rpi_2_model_b (Autodesk Fusion 360 design; units mm, degrees)
Autodesk Fusion 360 part; units mm, degrees
sketch "Sketch1" plane through (0, 0, 0) normal (0, 0, 1) x (1, 0, 0)
  line L0 (0, -3) -> (-79, -3)
  line L1 (-82, 0) -> (-82, 50)
  line L2 (-79, 53) -> (0, 53)
  line L3 (3, 50) -> (3, 0)
  arc A0 (-79, 53) -> (-82, 50) centre (-79, 50) ccw
  arc A1 (-82, 0) -> (-79, -3) centre (-79, 0) ccw
  arc A2 (3, 50) -> (0, 53) centre (0, 50) ccw
  arc A3 (0, -3) -> (3, 0) centre (0, 0) ccw
  circle A4 centre (-78.5, 49.5) radius 1.375
  circle A5 centre (-78.5, 0.5) radius 1.375
  circle A6 centre (-20.5, 49.5) radius 1.375
  circle A7 centre (-20.5, 0.5) radius 1.375
  dimension "d1" = 3
  dimension "d2" = 85
  dimension "d3" = 56
  dimension "d4" = 49
  dimension "d5" = 0.5
  dimension "d6" = 0.5
  dimension "d7" = 2.75
  dimension "d8" = 2.75
  dimension "d9" = 3.5
  dimension "d10" = 2.75
  dimension "d11" = 2.75
  dimension "d12" = 58
  dimension "d13" = 58
  dimension "d14" = 49
  dimension "d15" = 49
  constraint horizontal L0
  constraint vertical L1
  constraint horizontal L2
  constraint vertical L3
  constraint tangent L1 A0
  constraint tangent L2 A0
  constraint tangent L0 A1
  constraint tangent L1 A1
  constraint equal A0 A1
  constraint tangent L2 A2
  constraint tangent L3 A2
  constraint equal A0 A2
  constraint tangent L0 A3
  constraint tangent L3 A3
  constraint equal A0 A3
  constraint coincident A3.centre origin
  measures "d1" radius of A0
  measures "d2" distance of L1 L3
  measures "d3" distance of L0 L2
  measures "d4" distance of A4.centre A5.centre
  measures "d5" vertical distance of A0.centre A4.centre
  measures "d6" vertical distance of A1.centre A5.centre
  measures "d7" diameter of A4
  measures "d8" diameter of A5
  measures "d9" distance of L1 A5.centre
  measures "d10" diameter of A7
  measures "d11" diameter of A6
  measures "d12" horizontal distance of A4.centre A6.centre
  measures "d13" horizontal distance of A4.centre A7.centre
  measures "d14" vertical distance of A4.centre A7.centre
  measures "d15" vertical distance of A5.centre A6.centre
extrude "Extrude1" add sketch "Sketch1" along normal blind 1.6
sketch "Sketch2" plane through (0, 0, 0) normal (0, 0, -1) x (1, 0, 0)
  circle A0 centre (-20.5, -49.5) radius 1.375
  circle A1 centre (-78.5, -0.5) radius 1.375
  circle A2 centre (-20.5, -0.5) radius 1.375
  circle A3 centre (-78.5, -49.5) radius 1.375
  arc A4 (-79, 3) -> (-82, 0) centre (-79, 0) ccw
  line L0 (-82, 0) -> (-82, -50)
  arc A5 (-82, -50) -> (-79, -53) centre (-79, -50) ccw
  line L1 (-79, -53) -> (0, -53)
  arc A6 (0, -53) -> (3, -50) centre (0, -50) ccw
  line L2 (3, -50) -> (3, 0)
  arc A7 (3, 0) -> (0, 3) centre (0, 0) ccw
  line L3 (0, 3) -> (-79, 3)
  line L4 (-67.4, -18.5) -> (-85.4, -18.5)
  line L5 (-85.4, -18.5) -> (-85.4, -33.1)
  line L6 (-85.4, -33.1) -> (-67.4, -33.1)
  line L7 (-67.4, -33.1) -> (-67.4, -18.5)
  dimension "d18" = 14.6
  dimension "d19" = 19.9
  dimension "d20" = 18
  dimension "d21" = 3.4
  constraint horizontal L4
  constraint vertical L5
  constraint horizontal L6
  constraint vertical L7
  measures "d18" distance of L4.end L5.end
  measures "d19" distance of L1 L6
  measures "d20" distance of L4.start L4.end
  measures "d21" distance of L0 L5
extrude "Extrude2" add sketch "Sketch2" along normal blind 1.4 contours L0 L4 L6 L7 | L0 L4 L5 L6
extrude "Extrude3" add 1 faces at (-36.7049, 22.8333, 0) along direction (0, 0, -1) blind 2.45
sketch "Sketch3" plane through (0, 0, 1.6) normal (0, 0, 1) x (-1, 0, 0)
  circle A0 centre (20.5, -49.5) radius 1.375
  circle A1 centre (78.5, -0.5) radius 1.375
  circle A2 centre (20.5, -0.5) radius 1.375
  circle A3 centre (78.5, -49.5) radius 1.375
  arc A4 (82, 0) -> (79, 3) centre (79, 0) ccw
  line L0 (79, 3) -> (0, 3)
  arc A5 (0, 3) -> (-3, 0) centre (0, 0) ccw
  line L1 (-3, 0) -> (-3, -50)
  arc A6 (-3, -50) -> (0, -53) centre (0, -50) ccw
  line L2 (0, -53) -> (79, -53)
  arc A7 (79, -53) -> (82, -50) centre (79, -50) ccw
  line L3 (82, -50) -> (82, 0)
  line L4 (31.5, -9.5) -> (25.5, -9.5)
  line L5 (25.5, -9.5) -> (25.5, 3)
  line L6 (25.5, 3) -> (31.5, 3)
  line L7 (31.5, 3) -> (31.5, -9.5)
  line L8 (57.5, -7.1) -> (42.5, -7.1)
  line L9 (42.5, -7.1) -> (42.5, 4.5)
  line L10 (42.5, 4.5) -> (57.5, 4.5)
  line L11 (57.5, 4.5) -> (57.5, -7.1)
  line L12 (75.2, -1.2) -> (67.7, -1.2)
  line L13 (67.7, -1.2) -> (67.7, 4.5)
  line L14 (67.7, 4.5) -> (75.2, 4.5)
  line L15 (75.2, 4.5) -> (75.2, -1.2)
  dimension "d26" = 7.5
  dimension "d27" = 10.2
  dimension "d28" = 15
  dimension "d29" = 11
  dimension "d30" = 6
  dimension "d31" = 28.5
  dimension "d32" = 12.5
  dimension "d33" = 1.5
  dimension "d34" = 1.5
  dimension "d35" = 11.6
  dimension "d36" = 5.7
  constraint horizontal L4
  constraint vertical L5
  constraint horizontal L6
  constraint vertical L7
  constraint horizontal L8
  constraint vertical L9
  constraint horizontal L10
  constraint vertical L11
  constraint horizontal L12
  constraint vertical L13
  constraint horizontal L14
  constraint vertical L15
  constraint collinear L0 L6
  measures "d26" distance of L12.start L12.end
  measures "d27" distance of L11 L13
  measures "d28" distance of L8.start L8.end
  measures "d29" distance of L7 L9
  measures "d30" distance of L4.start L4.end
  measures "d31" distance of L1 L5
  measures "d32" distance of L4.start L6.end
  measures "d33" distance of L0 L10
  measures "d34" distance of L0 L14
  measures "d35" distance of L8.start L10.end
  measures "d36" distance of L12.end L13.end
extrude "Extrude4" add sketch "Sketch3" along normal blind 6.5 contours L0 L8 L9 L11 | L0 L9 L10 L11 | L0 L4 L5 L6 L7
extrude "Extrude5" add sketch "Sketch3" along normal blind 2.45 contours L0 L12 L13 L15 | L0 L13 L14 L15
sketch "Sketch4" plane through (0, -3, 0) normal (0, -1, 0) x (1, 0, 0)
  line L0 (0, -2.45) -> (0, 1.6)
  line L1 (0, 1.6) -> (-25.5, 1.6)
  line L2 (-25.5, 1.6) -> (-25.5, 8.1)
  line L3 (-25.5, 8.1) -> (-31.5, 8.1)
  line L4 (-31.5, 8.1) -> (-31.5, 1.6)
  line L5 (-31.5, 1.6) -> (-42.5, 1.6)
  line L6 (-42.5, 1.6) -> (-57.5, 1.6)
  line L7 (-57.5, 1.6) -> (-67.7, 1.6)
  line L8 (-67.7, 1.6) -> (-75.2, 1.6)
  line L9 (-75.2, 1.6) -> (-79, 1.6)
  line L10 (-79, 1.6) -> (-79, -2.45)
  line L11 (-79, -2.45) -> (0, -2.45)
  circle A0 centre (-28.5, 4.64) radius 3
  line L12 (-25.5, 1.6) -> (-31.5, 1.6)
  dimension "d41" = 6
  dimension "d42" = 3
  dimension "d43" = 3.04
  measures "d41" diameter of A0
  measures "d42" distance of L4 A0.centre
  measures "d43" distance of A0.centre L12
extrude "Extrude6" add sketch "Sketch4" along normal blind 2.5 contours A0
sketch "Sketch5" plane through (0, 0, 1.6) normal (0, 0, 1) x (1, 0, 0)
  line L0 (5.1, -0.25) -> (-16.3, -0.25)
  line L1 (-16.3, -0.25) -> (-16.3, 15.75)
  line L2 (-16.3, 15.75) -> (5.1, 15.75)
  line L3 (5.1, 15.75) -> (5.1, -0.25)
  line L4 (5.1, 19.75) -> (-12.1, 19.75)
  line L5 (-12.1, 19.75) -> (-12.1, 33.05)
  line L6 (-12.1, 33.05) -> (5.1, 33.05)
  line L7 (5.1, 33.05) -> (5.1, 19.75)
  line L8 (5.1, 37.55) -> (-12.1, 37.55)
  line L9 (-12.1, 37.55) -> (-12.1, 50.85)
  line L10 (-12.1, 50.85) -> (5.1, 50.85)
  line L11 (5.1, 50.85) -> (5.1, 37.55)
  line L12 (3, 0) -> (3, 50)
  line L13 (-79, -3) -> (0, -3)
  dimension "d46" = 13.3
  dimension "d47" = 13.3
  dimension "d48" = 16
  dimension "d49" = 2.1
  dimension "d50" = 2.1
  dimension "d51" = 2.1
  dimension "d52" = 4.5
  dimension "d53" = 4
  dimension "d54" = 2.75
  dimension "d55" = 21.4
  dimension "d56" = 17.2
  dimension "d57" = 17.2
  constraint horizontal L0
  constraint vertical L1
  constraint horizontal L2
  constraint vertical L3
  constraint horizontal L4
  constraint vertical L5
  constraint horizontal L6
  constraint vertical L7
  constraint horizontal L8
  constraint vertical L9
  constraint horizontal L10
  constraint vertical L11
  measures "d46" distance of L8.end L9.end
  measures "d47" distance of L4.end L5.end
  measures "d48" distance of L0.end L1.end
  measures "d49" distance of L3 L12
  measures "d50" distance of L7 L12
  measures "d51" distance of L11 L12
  measures "d52" distance of L6 L8
  measures "d53" distance of L2 L4
  measures "d54" distance of L0 L13
  measures "d55" distance of L1.end L2.end
  measures "d56" distance of L5.end L6.end
  measures "d57" distance of L9.end L10.end
extrude "Extrude7" add sketch "Sketch5" along normal blind 15.5 contours L4 L6 L7 L12 | L4 L5 L6 L12 | L8 L9 L10 L11
extrude "Extrude8" add sketch "Sketch5" along normal blind 13.8 contours L0 L1 L2 L3
sketch "Sketch6" plane through (0, 0, 1.6) normal (0, 0, 1) x (-1, 0, 0)
  line L0 (16.3, -15.75) -> (-3, -15.75)
  line L1 (-3, -15.75) -> (-3, -19.75)
  line L2 (-3, -19.75) -> (12.1, -19.75)
  line L3 (12.1, -19.75) -> (12.1, -33.05)
  line L4 (12.1, -33.05) -> (-3, -33.05)
  line L5 (-3, -33.05) -> (-3, -37.55)
  line L6 (-3, -37.55) -> (12.1, -37.55)
  line L7 (12.1, -37.55) -> (12.1, -50.85)
  line L8 (12.1, -50.85) -> (-2.8771, -50.85)
  arc A0 (-2.8771, -50.85) -> (0, -53) centre (0, -50) ccw
  line L9 (0, -53) -> (79, -53)
  arc A1 (79, -53) -> (82, -50) centre (79, -50) ccw
  line L10 (82, -50) -> (82, 0)
  arc A2 (82, 0) -> (79, 3) centre (79, 0) ccw
  line L11 (79, 3) -> (75.2, 3)
  line L12 (75.2, 3) -> (75.2, -1.2)
  line L13 (75.2, -1.2) -> (67.7, -1.2)
  line L14 (67.7, -1.2) -> (67.7, 3)
  line L15 (67.7, 3) -> (57.5, 3)
  line L16 (57.5, 3) -> (57.5, -7.1)
  line L17 (57.5, -7.1) -> (42.5, -7.1)
  line L18 (42.5, -7.1) -> (42.5, 3)
  line L19 (42.5, 3) -> (31.5, 3)
  line L20 (31.5, 3) -> (31.5, -9.5)
  line L21 (31.5, -9.5) -> (25.5, -9.5)
  line L22 (25.5, -9.5) -> (25.5, 3)
  line L23 (25.5, 3) -> (0, 3)
  arc A3 (0, 3) -> (-2.9896, 0.25) centre (0, 0) ccw
  line L24 (-2.9896, 0.25) -> (16.3, 0.25)
  line L25 (16.3, 0.25) -> (16.3, -15.75)
  circle A4 centre (20.5, -49.5) radius 1.375
  circle A5 centre (78.5, -0.5) radius 1.375
  circle A6 centre (20.5, -0.5) radius 1.375
  circle A7 centre (78.5, -49.5) radius 1.375
  line L26 (75.2, -51.94) -> (24.2, -51.94)
  line L27 (24.2, -51.94) -> (24.2, -46.94)
  line L28 (24.2, -46.94) -> (75.2, -46.94)
  line L29 (75.2, -46.94) -> (75.2, -51.94)
  dimension "d62" = 6.8
  dimension "d63" = 1.06
  dimension "d64" = 51
  dimension "d65" = 5
  constraint horizontal L26
  constraint vertical L27
  constraint horizontal L28
  constraint vertical L29
  measures "d62" distance of L10 L29
  measures "d63" distance of L9 L26
  measures "d64" distance of L26.start L26.end
  measures "d65" distance of L26.start L28.end
extrude "Extrude9" add sketch "Sketch6" along normal blind 8.1 contours L26 L27 L28 L29
sketch "Sketch7" plane through (0, 0, 1.6) normal (0, 0, 1) x (-1, 0, 0)
  line L0 (75.2, -46.94) -> (75.2, -51.94)
  line L1 (75.2, -51.94) -> (24.2, -51.94)
  line L2 (24.2, -51.94) -> (24.2, -46.94)
  line L3 (24.2, -46.94) -> (75.2, -46.94)
  line L4 (16.3, -15.75) -> (-3, -15.75)
  line L5 (-3, -15.75) -> (-3, -19.75)
  line L6 (-3, -19.75) -> (12.1, -19.75)
  line L7 (12.1, -19.75) -> (12.1, -33.05)
  line L8 (12.1, -33.05) -> (-3, -33.05)
  line L9 (-3, -33.05) -> (-3, -37.55)
  line L10 (-3, -37.55) -> (12.1, -37.55)
  line L11 (12.1, -37.55) -> (12.1, -50.85)
  line L12 (12.1, -50.85) -> (-2.8771, -50.85)
  arc A0 (-2.8771, -50.85) -> (0, -53) centre (0, -50) ccw
  line L13 (0, -53) -> (79, -53)
  arc A1 (79, -53) -> (82, -50) centre (79, -50) ccw
  line L14 (82, -50) -> (82, 0)
  arc A2 (82, 0) -> (79, 3) centre (79, 0) ccw
  line L15 (79, 3) -> (75.2, 3)
  line L16 (75.2, 3) -> (75.2, -1.2)
  line L17 (75.2, -1.2) -> (67.7, -1.2)
  line L18 (67.7, -1.2) -> (67.7, 3)
  line L19 (67.7, 3) -> (57.5, 3)
  line L20 (57.5, 3) -> (57.5, -7.1)
  line L21 (57.5, -7.1) -> (42.5, -7.1)
  line L22 (42.5, -7.1) -> (42.5, 3)
  line L23 (42.5, 3) -> (31.5, 3)
  line L24 (31.5, 3) -> (31.5, -9.5)
  line L25 (31.5, -9.5) -> (25.5, -9.5)
  line L26 (25.5, -9.5) -> (25.5, 3)
  line L27 (25.5, 3) -> (0, 3)
  arc A3 (0, 3) -> (-2.9896, 0.25) centre (0, 0) ccw
  line L28 (-2.9896, 0.25) -> (16.3, 0.25)
  line L29 (16.3, 0.25) -> (16.3, -15.75)
  circle A4 centre (20.5, -49.5) radius 1.375
  circle A5 centre (78.5, -0.5) radius 1.375
  circle A6 centre (20.5, -0.5) radius 1.375
  circle A7 centre (78.5, -49.5) radius 1.375
  line L30 (62, -35.5) -> (48, -35.5)
  line L31 (48, -35.5) -> (48, -21.5)
  line L32 (48, -21.5) -> (62, -21.5)
  line L33 (62, -21.5) -> (62, -35.5)
  line L34 (79, -53) -> (0, -53)
  line L35 (82, 0) -> (82, -50)
  dimension "d68" = 31.5
  dimension "d69" = 34
  dimension "d70" = 14
  dimension "d71" = 14
  constraint horizontal L30
  constraint vertical L31
  constraint horizontal L32
  constraint vertical L33
  measures "d68" distance of L32 L34
  measures "d69" distance of L31 L35
  measures "d70" distance of L31.end L32.end
  measures "d71" distance of L30.end L31.end
extrude "Extrude10" add sketch "Sketch7" along normal blind 1 contours L30 L31 L32 L33
equation "d8 = d7"
equation "d10 = d7"
equation "d11 = d7"
equation "d13 = d12"
equation "d14 = d4"
equation "d15 = d4"
equation "d21 = d20 - 14.6 mm"
equation "d47 = d46"
equation "d50 = d49"
equation "d51 = d49"
equation "d57 = d56"
